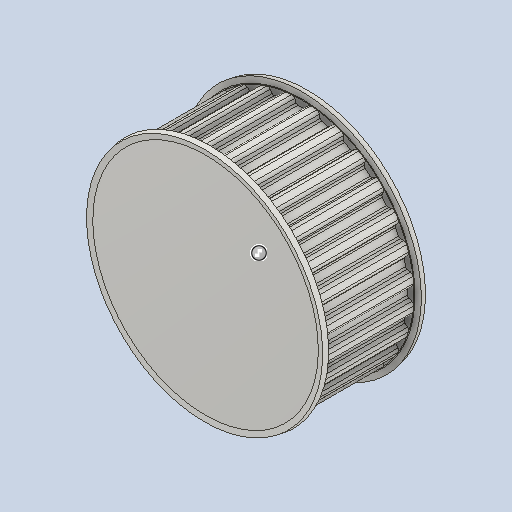
# Autodesk Inventor part: Synchroniczne koło pasowe3
Saved by Autodesk Inventor 2023 (Build 270158000, 158)
## iProperties
CustomPartVersion: 1
Created: 2023-05-15
Part Number: Synchroniczne koło pasowe3
Material: Steel
Document SubType Name: Modeling
Designer: krzys
Density: 7.85 g/cm^3
Appearance: Steel
Mass: 219.222 g
Surface Area: 70.5623 cm^2
Volume: 27.9263 cm^3
Author: krzys
Autodesk Inventor part; units mm, degrees
ref_plane "YZ Plane" through (0, 0, 0) normal (1, 0, 0) x (0, 1, 0)
ref_plane "XZ Plane" through (0, 0, 0) normal (0, 1, 0) x (-1, 0, 0)
ref_plane "XY Plane" through (0, 0, 0) normal (0, 0, 1) x (1, 0, 0)
sketch "Szkic koła pasowego" plane through (0, 0, 0) normal (0, 0, 1) x (1, 0, 0)
  circle A0 centre (0, 0) radius 22.2817 construction
  circle A1 centre (0, 0) radius 21.7817
  circle A2 centre (0, 0) radius 20.5317
  line L0 (-1.46, 21.7327) -> (-0.9, 20.5317)
  line L1 (-0.9, 20.5317) -> (0.9, 20.5317)
  line L2 (0.9, 20.5317) -> (1.46, 21.7327)
  line L3 (0, 0) -> (0, 21.7817) construction
  point P0 (0, 20.5317)
  dimension "d0" = 44.5634
  dimension "d1" = 0.5
  dimension "d2" = 1.25
  dimension "d3" = 50
  dimension "d4" = 1.8
  constraints: 8 end point, 3 coincident, 3 point on circle, 2 centre point, 1 horizontal, 1 midpoint, 1 point on line, 1 vertical, 1 vertical alignment, 3 other
  measures "d0" diameter of A0
  measures "d1" radial gap between concentric circles of A0 A1
  measures "d3" angle of L2 L0
  measures "d4" distance of L0.end L1.end
extrude "Bryła podstawowa" add sketch "Szkic koła pasowego" along normal mid plane 17.5 contours A2 | A1 L0 L1 L2 | L2 L1 L0 A1
extrude "Ząb" cut sketch "Szkic koła pasowego" along normal through all both and the other way through all contours L2 L1 L0 A1 picked at (0, 21.3614)
fillet "Fillet" radius 0.4 2 edges at (0.9, 20.5317, 0) (-0.9, 20.5317, 0)
fillet "Fillet" radius 0.6 4 edges at (-1.46, 21.7327, 4.375) (-1.46, 21.7327, -4.375) (1.46, 21.7327, 4.375) (1.46, 21.7327, -4.375)
pattern_circular "Zęby" count 28 over 360 about axis through (0, 0, -10) along (0, 0, 1) of "Ząb", "Fillet"
pulley flange "Obrzeże lewe" diameter 43.5634 height 1.2 thickness 1 bend angle 10 centre (0, 0, -8.75) toward (0, 0, -1)
pulley flange "Obrzeże prawe" diameter 43.5634 height 1.2 thickness 1 bend angle 10 centre (0, 0, 8.75) toward (0, 0, 1)
equation "\"d1\" = da_a"
equation "\"d2\" = da_hg"
equation "\"d3\" = 2 * da_fi"
equation "\"d4\" = da_bw"
equation "\"d5\" = da_bf"
equation "\"d7\" = da_bf"
equation "\"d9\" = da_rb"
equation "\"d10\" = da_rt"
equation "\"da_pb\" = 5"
equation "\"da_fi\" = 25deg"
equation "\"da_hg\" = 1.25"
equation "\"da_bw\" = 1.8"
equation "\"da_rb\" = 0.4"
equation "\"da_rt\" = 0.6"
equation "\"da_a\" = 0.5"
equation "\"da_bf\" = 17.5"
equation "\"da_wf\" = 1"
equation "\"da_hf\" = 1.2"
body "Solid1"
